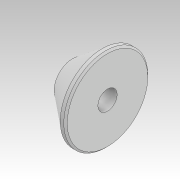
# Autodesk Inventor part: BaseWasher
Saved by Autodesk Inventor 2020 (Build 240168000, 168)
## iProperties
Created: 2022-09-05
Part Number: BaseWasher
Material: Generic
Document SubType Name: Modeling
Designer: DDeGo
Density: 1 g/cm^3
Appearance: Default
Author: DDeGo
Autodesk Inventor part; units mm, degrees
ref_plane "YZ Plane" through (0, 0, 0) normal (1, 0, 0) x (0, 1, 0)
ref_plane "XZ Plane" through (0, 0, 0) normal (0, 1, 0) x (-1, 0, 0)
ref_plane "XY Plane" through (0, 0, 0) normal (0, 0, 1) x (1, 0, 0)
sketch "Sketch1" plane through (0, 0, 0) normal (0, 0, 1) x (1, 0, 0)
  line L0 (0, 0) -> (-10, 0) construction
  line L1 (-10, 0) -> (-10, 2.75) construction
  line L2 (-10, 2.75) -> (0, 2.75)
  line L3 (0, 2.75) -> (0, 0) construction
  line L4 (0, 2.75) -> (0, 11.5)
  line L5 (-0.5, 12) -> (-1.5, 12)
  line L6 (-1.5, 12) -> (-10, 5.25)
  line L7 (-10, 5.25) -> (-10, 2.75)
  line L8 (-0.5, 12) -> (0, 11.5)
  point P0 (0, 12)
  dimension "d0" = 2.75
  dimension "d1" = 10
  dimension "d2" = 2.5
  dimension "d3" = 1.5
  dimension "d4" = 12
  dimension "d5" = 0.5
  dimension "d6" = 0.5
  constraints: 18 end point, 5 perpendicular, 4 point on line, 1 horizontal
  measures "d0" distance between parallel lines of L0 L2
  measures "d1" distance of L0.start L0.end
  measures "d2" distance of L6.end L1.end
  measures "d3" distance of point (0, 12) L5.end
  measures "d4" distance between parallel lines of L0 L5
  measures "d5" distance of L5.start point (0, 12)
  measures "d6" distance of L4.end point (0, 12)
revolve "Revolution1" add sketch "Sketch1" angle 360 about axis through (0, 0, 0) along (-1, 0, 0)
equation "\"d6\" = d5"
body "Solid1"
